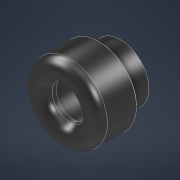
# Autodesk Inventor part: cap_top
Saved by Autodesk Inventor 2022.1 (Build 261234020, 234B)
## iProperties
Created: 2021-12-02
Part Number: cap_top
Material: Generic
Document SubType Name: Modeling
Designer: PaulT
Density: 1 g/cm^3
Appearance: Glossy - Black
Author: PaulT
Autodesk Inventor part; units mm, degrees
ref_plane "YZ Plane" through (0, 0, 0) normal (1, 0, 0) x (0, 1, 0)
ref_plane "XZ Plane" through (0, 0, 0) normal (0, 1, 0) x (-1, 0, 0)
ref_plane "XY Plane" through (0, 0, 0) normal (0, 0, 1) x (1, 0, 0)
sketch "Sketch1" plane through (0, 0, 0) normal (0, 0, 1) x (1, 0, 0)
  circle A0 centre (0, 0) radius 4.85
  dimension "d0" = 9.7
  constraints: 1 centre point, 1 coincident
  measures "d0" diameter of A0
extrude "Extrusion1" add sketch "Sketch1" against normal blind 7.84
sketch "Sketch2" plane through (0, 0, -7.84) normal (0, 0, -1) x (-1, 0, 0)
  circle A0 centre (0, 0) radius 4.85
  circle A1 centre (0, 0) radius 3.65
  circle A2 centre (0, 0) radius 4.85 projected
  dimension "d3" = 7.3
  constraints: 2 centre point, 2 coincident, 1 concentric
  measures "d3" diameter of A1
extrude "Extrusion2" cut sketch "Sketch2" against normal blind 2.6
sketch "Sketch5" plane through (0, 0, -7.84) normal (0, 0, -1) x (-1, 0, 0)
  circle A0 centre (0, 0) radius 2.7
  dimension "d21" = 5.4
  constraints: 1 centre point, 1 coincident
  measures "d21" diameter of A0
extrude "Extrusion4" cut sketch "Sketch5" against normal blind 6
sketch "Sketch6" plane through (0, 0, -1.84) normal (0, 0, -1) x (-1, 0, 0)
  circle A0 centre (0, 0) radius 2.25
  dimension "d24" = 4.5
  constraints: 1 centre point, 1 coincident
  measures "d24" diameter of A0
extrude "Extrusion5" cut sketch "Sketch6" against normal through all
sketch "Sketch7" plane through (0, 0, 0) normal (1, 0, 0) x (0, 1, 0)
  line L0 (4.85, 1) -> (4.85, -1.3)
  arc A0 (4.85, -1.3) -> (2.25, -1.3) centre (3.55, -1.3) ccw
  line L1 (2.25, -1.3) -> (2.25, 1)
  line L2 (2.25, 1) -> (4.85, 1)
  line L3 (0, 6.9365) -> (0, -11.7629) construction
  point P0 (0, 0)
  point P1 (4.85, -0.15)
  dimension "d27" = 4.85
  dimension "d28" = 2.25
  dimension "d29" = 1.3
  dimension "d30" = 1
  constraints: 8 end point, 2 point on circle, 2 tangent, 2 vertical, 1 centre point, 1 midpoint, 1 parallel, 1 perpendicular
  measures "d27" horizontal distance of point (0, 0) point (4.85, -0.15)
  measures "d28" distance from line of point (0, 0) L1
  measures "d29" vertical distance of point (0, 0) A0.centre
  measures "d30" distance from line of point (0, 0) L2
revolve "Revolution2" cut sketch "Sketch7" angle 360 about axis through (0, 0, 6.9365) along (0, 0, -1)
chamfer "Chamfer2" distance 0.2 angle 45 1 edges at (-4.85, 0, -5.24)
body "Solid1"
